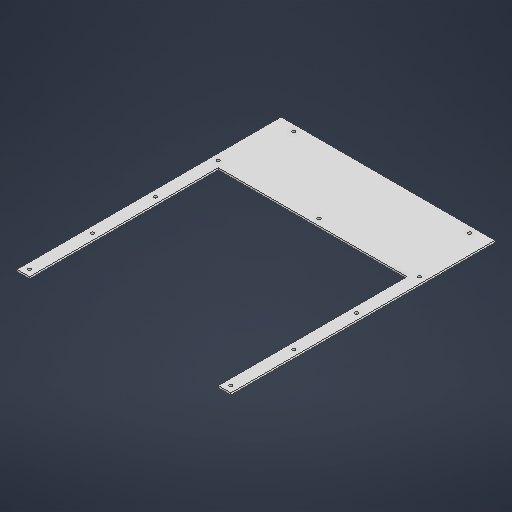
# Autodesk Inventor part: CaraFrontal
Saved by Autodesk Inventor 2026.2 (Build 302298010, 298A)
## iProperties
Created: 2026-04-15
Part Number: CaraFrontal
Material: Generic
Document SubType Name: Modeling
Designer: grego
Density: 1 g/cm^3
Appearance: Default
Author: grego
Autodesk Inventor part; units mm, degrees
ref_plane "YZ Plane" through (0, 0, 0) normal (1, 0, 0) x (0, 1, 0)
ref_plane "XZ Plane" through (0, 0, 0) normal (0, 1, 0) x (-1, 0, 0)
ref_plane "XY Plane" through (0, 0, 0) normal (0, 0, 1) x (1, 0, 0)
sketch "Sketch1" plane through (0, 0, 0) normal (0, 1, 0) x (-1, 0, 0)
  line L0 (190, 210) -> (190, -210)
  line L1 (190, -210) -> (-150, -210)
  line L2 (-150, -210) -> (-150, 210)
  line L3 (-150, -190) -> (170, -190)
  line L4 (170, -190) -> (170, 190)
  line L5 (-150, -200) -> (180, -200)
  line L6 (180, -200) -> (180, 200)
  line L7 (190, -210) -> (190, -90)
  line L8 (190, -90) -> (-150, -90)
  line L9 (170, 190) -> (170, 210)
  line L10 (180, 200) -> (180, 210)
  line L11 (170, 210) -> (190, 210)
  line L12 (190, -90) -> (190, -100)
  line L13 (190, -100) -> (-150, -100)
  line L14 (190, -100) -> (190, -110)
  line L15 (190, -110) -> (-150, -110)
  circle A0 centre (180, 200) radius 2.5
  circle A1 centre (180, -100) radius 2.5
  circle A2 centre (20, -100) radius 2.5
  circle A3 centre (180, 100) radius 2.5
  circle A4 centre (180, 0) radius 2.5
  line L16 (0, 0) -> (0, 25.5231)
  circle A5 centre (160, -200) radius 2.5
  line L17 (-150, -200) -> (-140, -200)
  line L18 (-140, -200) -> (-130, -200)
  line L19 (-130, -200) -> (-130, 210)
  line L20 (-130, 210) -> (-150, 210)
  circle A6 centre (-140, -100) radius 2.5
  circle A7 centre (-140, 0) radius 2.5
  circle A8 centre (-140, 100) radius 2.5
  circle A9 centre (-140, 200) radius 2.5
  circle A10 centre (20, -200) radius 2.5
  line L21 (20, -200) -> (-120, -200)
  circle A11 centre (-120, -200) radius 2.5
  point P0 (170, -90)
  point P1 (180, -90)
  point P2 (-130, -90)
  point P3 (-130, -190)
  point P4 (180, 2.5)
  point P5 (180, -2.5)
  point P6 (180, 202.5)
  point P7 (180, 197.5)
  point P8 (180, 102.5)
  point P9 (180, 97.5)
  dimension "d0" = 340
  dimension "d1" = 420
  dimension "d2" = 20
  dimension "d3" = 10
  dimension "d4" = 120
  dimension "d5" = 10
  dimension "d6" = 10
  dimension "d7" = 5
  dimension "d9" = 5
  dimension "d11" = 5
  dimension "d12" = 5
  dimension "d13" = 5
  dimension "d15" = 5
  dimension "d25" = 10
  dimension "d26" = 10
  dimension "d27" = 5
  dimension "d30" = 5
  dimension "d31" = 140
  dimension "d32" = 5
  constraints: 44 end point, 17 point on line, 12 centre point, 7 perpendicular, 3 midpoint, 3 parallel, 2 coincident, 1 horizontal, 1 vertical
  measures "d0" distance of L0.end L1.end
  measures "d1" distance of L0.start L0.end
  measures "d2" distance between parallel lines of L1 L3
  measures "d3" distance between parallel lines of L1 L5
  measures "d4" distance of L0.end L7.end
  measures "d5" distance of L7.end L12.end
  measures "d6" distance of L12.end L14.end
  measures "d7" diameter of A0
  measures "d9" diameter of A1
  measures "d11" diameter of A2
  measures "d12" diameter of A3
  measures "d13" diameter of A4
  measures "d15" diameter of A5
  measures "d25" distance of L5.start L17.end
  measures "d26" distance of L17.end L18.end
  measures "d27" diameter of A7
  measures "d30" diameter of A10
  measures "d31" distance of L21.start L21.end
  measures "d32" diameter of A11
extrude "Extrusion1" add sketch "Sketch1" along normal blind 3 contours L0 L8 L6 A4 A3 A0 L10 L11 | L0 L13 A1 L6 L8 | L10 A0 L6 A3 A4 L8 L4 L9 L11 | L0 L15 L6 A1 L13 | L6 A1 L13 L4 L8 | L0 L1 L2 L5 A11 A10 A5 L6 L15 | L4 L13 A2 L19 L8 | L15 L4 L13 A1 L6 | L6 L5 A5 A10 A11 L19 L3 L4 L15 | L4 L15 L19 L13 A2 | L19 L13 A6 L2 L8 | L8 L2 L20 L19 | L4 L3 L19 L15 | L19 L15 L2 L13 A6 | L2 L3 L19 L5 | L19 L3 L2 L15 | A6 L13 | L13 A6 | A10 L5 | L5 A10 | A11 L5 | L5 A11
sketch "Sketch3" plane through (0, 3, 0) normal (0, 1, 0) x (1, 0, 0)
  circle A0 centre (-180, -100) radius 2.5 projected
  circle A1 centre (-20, 100) radius 2.5 projected
  circle A2 centre (-160, 200) radius 2.5 projected
  circle A3 centre (-180, 100) radius 2.5 projected
  circle A4 centre (140, 0) radius 2.5 projected
  circle A5 centre (140, -100) radius 2.5 projected
  circle A6 centre (140, -200) radius 2.5 projected
  circle A7 centre (-180, -200) radius 2.5 projected
  line L0 (-190, 210) -> (-190, -210) projected
  line L1 (-190, -210) -> (-170, -210) projected
  line L2 (-170, -210) -> (-170, 90) projected
  line L3 (-170, 90) -> (130, 90) projected
  line L4 (130, 90) -> (130, -210) projected
  line L5 (130, -210) -> (150, -210) projected
  line L6 (150, -210) -> (150, 210) projected
  line L7 (150, 210) -> (-190, 210) projected
  circle A8 centre (-180, 0) radius 2.5 projected
  circle A9 centre (-20, 200) radius 2.5 projected
  circle A10 centre (120, 200) radius 2.5 projected
  circle A11 centre (-180, -100) radius 2.5 projected
  circle A12 centre (-20, 100) radius 2.5 projected
  circle A13 centre (-160, 200) radius 2.5 projected
  circle A14 centre (-180, 100) radius 2.5 projected
  circle A15 centre (140, 0) radius 2.5 projected
  circle A16 centre (140, -100) radius 2.5 projected
  circle A17 centre (140, -200) radius 2.5 projected
  circle A18 centre (-180, -200) radius 2.5 projected
  line L8 (-190, 210) -> (-190, -210) projected
  line L9 (-190, -210) -> (-170, -210) projected
  line L10 (-170, -210) -> (-170, 90) projected
  line L11 (-170, 90) -> (130, 90) projected
  line L12 (130, 90) -> (130, -210) projected
  line L13 (130, -210) -> (150, -210) projected
  line L14 (150, -210) -> (150, 210) projected
  line L15 (150, 210) -> (-190, 210) projected
  circle A19 centre (-180, 0) radius 2.5 projected
  circle A20 centre (140, 100) radius 2.5 projected
  point P0 (0, 0)
extrude "Extrusion3" cut sketch "Sketch3" against normal blind 3 contours A10 | A20
body "Solid1"
